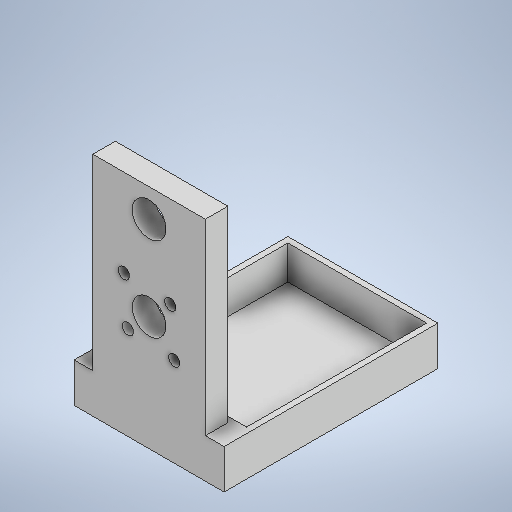
# Autodesk Inventor part: Motor Stand
Saved by Autodesk Inventor 2026.1 (Build 301233020, 233B)
## iProperties
Created: 2025-10-20
Part Number: Motor Stand
Material: Generic
Document SubType Name: Modeling
Designer: yo
Density: 1 g/cm^3
Appearance: Default
Author: yo
Autodesk Inventor part; units mm, degrees
ref_plane "YZ Plane" through (0, 0, 0) normal (1, 0, 0) x (0, 1, 0)
ref_plane "XZ Plane" through (0, 0, 0) normal (0, 1, 0) x (-1, 0, 0)
ref_plane "XY Plane" through (0, 0, 0) normal (0, 0, 1) x (1, 0, 0)
sketch "Sketch1" plane through (0, 0, 0) normal (0, 1, 0) x (-1, 0, 0)
  line L0 (18.5, -24) -> (-18.5, -24)
  line L1 (-18.5, -24) -> (-18.5, 24)
  line L2 (-18.5, 24) -> (18.5, 24)
  line L3 (18.5, 24) -> (18.5, -24)
  line L4 (20, -25.5) -> (-20, -25.5)
  line L5 (-20, -25.5) -> (-20, 25.5)
  line L6 (-20, 25.5) -> (20, 25.5)
  line L7 (20, 25.5) -> (20, -25.5)
  point P0 (0, 0)
  point P1 (0, -24)
  point P2 (-18.5, 0)
  point P3 (-20, 0)
  point P4 (0, -25.5)
  dimension "d0" = 37
  dimension "d1" = 48
  dimension "d2" = 1.5
  dimension "d3" = 1.5
  constraints: 16 end point, 4 midpoint, 4 parallel, 2 horizontal, 2 horizontal alignment, 2 perpendicular, 2 vertical alignment
  measures "d0" distance of L0.start L0.end
  measures "d1" distance of L0.end L1.end
  measures "d2" distance between parallel lines of L5 L1
  measures "d3" distance between parallel lines of L0 L4
extrude "Extrusion1" add sketch "Sketch1" along normal blind 9
extrude "Extrusion2" add sketch "Sketch1" against normal blind 1.5 contours L0 L1 L2 L3 | L4 L5 L6 L7
sketch "Sketch2" plane through (-20, 9, 25.5) normal (0, 0, 1) x (1, 0, 0)
  line L0 (5, 35) -> (35, 35) construction
  line L1 (35, 35) -> (35, 5)
  line L2 (35, 5) -> (5, 5) construction
  line L3 (5, 5) -> (5, 35)
  circle A0 centre (20, 20) radius 4.5
  circle A1 centre (14.3431, 14.3431) radius 1.5
  circle A2 centre (13.2825, 26.7175) radius 1.5
  circle A3 centre (25.6569, 25.6569) radius 1.5
  circle A4 centre (26.7175, 13.2825) radius 1.5
  line L4 (14.3431, 14.3431) -> (25.6569, 25.6569) construction
  line L5 (13.2825, 26.7175) -> (26.7175, 13.2825) construction
  line L6 (0, 0) -> (40, 0) projected
  line L7 (25.6569, 25.6569) -> (35, 35) construction
  line L8 (40, -10.5) -> (40, 0) projected
  line L9 (0, 0) -> (40, 0) projected
  line L10 (0, 0) -> (0, -10.5) projected
  line L11 (40, -10.5) -> (0, -10.5) projected
  circle A5 centre (20, 20) radius 13.9 construction
  line L12 (5, 5) -> (5, 0)
  line L13 (35, 5) -> (35, 0)
  circle A6 centre (20, 42.5) radius 4.5
  line L14 (5, 35) -> (5, 50)
  line L15 (5, 50) -> (35, 50)
  line L16 (35, 50) -> (35, 35)
  point P0 (20, -9)
  point P1 (20, 35)
  point P2 (35, 20)
  point P3 (20, 5)
  point P4 (20, 0)
  point P5 (5, 0)
  point P6 (35, 0)
  point P7 (5, 0)
  point P8 (35, 0)
  dimension "d8" = 9
  dimension "d9" = 3
  dimension "d10" = 16
  dimension "d11" = 19
  dimension "d12" = 30
  dimension "d16" = 27.8
  dimension "d17" = 5
  dimension "d19" = 7.5
  dimension "d20" = 15
  constraints: 24 end point, 7 centre point, 6 midpoint, 6 perpendicular, 4 coincident, 4 equal radius, 3 vertical alignment, 2 parallel, 2 point on line, 2 vertical, 1 collinear, 1 horizontal, 1 horizontal alignment
  measures "d8" diameter of A0
  measures "d9" diameter of A1
  measures "d10" distance of L4.start L4.end
  measures "d11" distance of L5.start L5.end
  measures "d12" distance of L0.end L1.end
  measures "d16" diameter of A5
  measures "d17" distance between parallel lines of L9 L2
  measures "d19" distance from line of L0 A6.centre
  measures "d20" distance of L15.end L0.end
extrude "Extrusion3" add sketch "Sketch2" along normal blind 6
equation "\"d20\" = 2 * d19"
body "Solid1"
